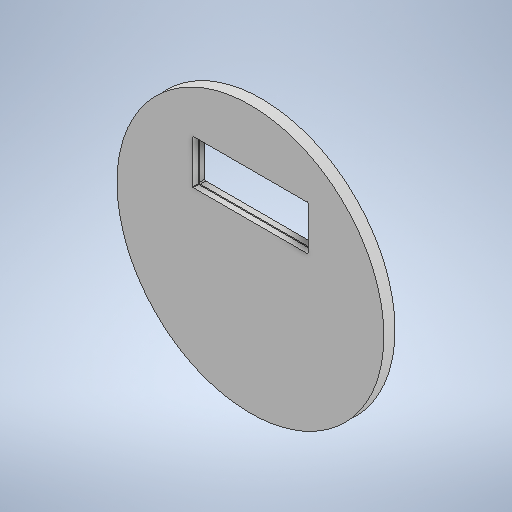
# Autodesk Inventor part: Base Plate
Saved by Autodesk Inventor 2025.2 (Build 292293000, 293)
## iProperties
Created: 2025-06-01
Part Number: Base Plate
Material: Generic
Document SubType Name: Modeling
Designer: dylan
Density: 1 g/cm^3
Appearance: Default
Author: dylan
Autodesk Inventor part; units mm, degrees
ref_plane "YZ Plane" through (0, 0, 0) normal (1, 0, 0) x (0, 1, 0)
ref_plane "XZ Plane" through (0, 0, 0) normal (0, 1, 0) x (-1, 0, 0)
ref_plane "XY Plane" through (0, 0, 0) normal (0, 0, 1) x (1, 0, 0)
sketch "Sketch1" plane through (0, 0, 0) normal (0, 0, 1) x (1, 0, 0)
  circle A0 centre (0, 0) radius 600
  circle A1 centre (0, 0) radius 575
  circle A2 centre (0, 0) radius 525
  dimension "d0" = 1200
  dimension "d3" = 1150
  dimension "d4" = 1050
  constraints: 3 centre point, 3 coincident
  measures "d0" diameter of A0
  measures "d3" diameter of A1
  measures "d4" diameter of A2
extrude "Extrusion1" add sketch "Sketch1" along normal blind 50 contours A0 | A1 | A2
extrude "Extrusion2" cut sketch "Sketch1" along normal blind 20 contours A1
sketch "Sketch2" plane through (0, 0, 50) normal (0, 0, 1) x (1, 0, 0)
  line L0 (0, 0) -> (0, 350) construction
  line L1 (0, 350) -> (-255.3075, 350) construction
  line L2 (-259.8075, 350) -> (255.3075, 350)
  line L3 (259.8075, 345.5) -> (259.8075, 154.5)
  line L4 (255.3075, 150) -> (-257.8075, 150)
  line L5 (-259.8075, 152) -> (-259.8075, 345.5)
  arc A0 (-259.8075, 152) -> (-257.8075, 150) centre (-257.8075, 152) ccw
  arc A1 (-255.3075, 350) -> (-259.8075, 345.5) centre (-255.3075, 345.5) ccw
  arc A2 (259.8075, 345.5) -> (255.3075, 350) centre (255.3075, 345.5) ccw
  arc A3 (255.3075, 150) -> (259.8075, 154.5) centre (255.3075, 154.5) ccw
  line L6 (-259.8075, 150) -> (-259.8075, 154.5) construction
  line L7 (-259.8075, 154.5) -> (-255.3075, 154.5) construction
  line L8 (255.3075, 350) -> (255.3075, 345.5) construction
  line L9 (250.8075, 345.5) -> (-250.8075, 345.5)
  line L10 (-255.3075, 341) -> (-255.3075, 159)
  line L11 (-250.8075, 154.5) -> (250.8075, 154.5)
  line L12 (255.3075, 159) -> (255.3075, 341)
  arc A4 (-255.3075, 159) -> (-250.8075, 154.5) centre (-250.8075, 159) ccw
  arc A5 (-250.8075, 345.5) -> (-255.3075, 341) centre (-250.8075, 341) ccw
  arc A6 (255.3075, 341) -> (250.8075, 345.5) centre (250.8075, 341) ccw
  arc A7 (250.8075, 154.5) -> (255.3075, 159) centre (250.8075, 159) ccw
  point P0 (259.8075, 350)
  dimension "d7" = 350
  dimension "d8" = 259.8075
  dimension "d9" = 519.615
  dimension "d10" = 200
  dimension "d11" = 2
  dimension "d12" = 4.5
  dimension "d13" = 4.5
  dimension "d14" = 4.5
  dimension "d15" = 4.5
  constraints: 26 end point, 16 point on circle, 16 tangent, 11 point on line, 8 centre point, 5 equal radius, 4 horizontal, 4 parallel, 2 perpendicular, 2 vertical
  measures "d7" distance of L0.start L0.end
  measures "d8" distance of L0.end L2.start
  measures "d9" distance of L2.start point (259.808, 350)
  measures "d10" distance of L6.start L2.start
  measures "d11" radius of A0
  measures "d12" radius of A1
  measures "d13" distance of L6.start L6.end
  measures "d14" distance of L6.end L7.end
  measures "d15" radius of A4
extrude "Extrusion3" cut sketch "Sketch2" against normal through all contours A6 L12 A7 L11 A4 L10 A5 L9
extrude "Extrusion4" cut sketch "Sketch2" against normal blind 25
body "Solid1"
